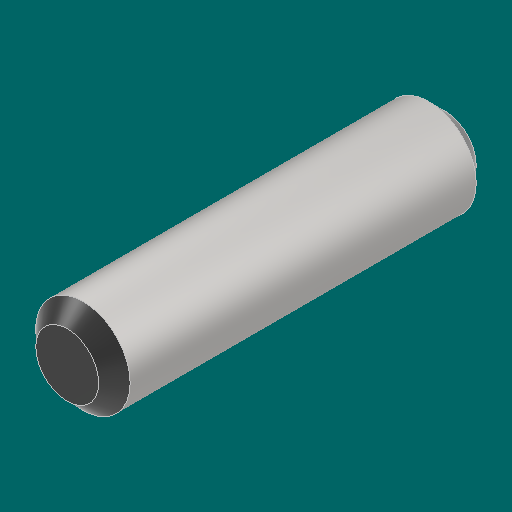
# Autodesk Inventor part: HeikoPin
Saved by Autodesk Inventor 2023 (Build 270158000, 158)
## iProperties
Created: 2022-03-28
Part Number: HeikoPin
Material: 一般
Document SubType Name: Modeling
Designer: neko2
Density: 1 g/cm^3
Appearance: 既定
Author: neko2
Autodesk Inventor part; units mm, degrees
ref_plane "YZ Plane" through (0, 0, 0) normal (1, 0, 0) x (0, 1, 0)
ref_plane "XZ Plane" through (0, 0, 0) normal (0, 1, 0) x (-1, 0, 0)
ref_plane "XY Plane" through (0, 0, 0) normal (0, 0, 1) x (1, 0, 0)
sketch "スケッチ1" plane through (0, 0, 0) normal (0, 0, 1) x (1, 0, 0)
  circle A0 centre (0, 0) radius 1.5
  dimension "d0" = 3
  constraints: 1 centre point, 1 coincident
  measures "d0" diameter of A0
extrude "押し出し1" add sketch "スケッチ1" along normal blind 12
chamfer "面取り1" distance 0.5 angle 45 2 edges at (-1.5, 0, 12) (-1.5, 0, 0)
